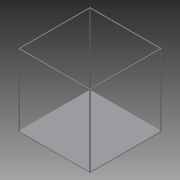
# Autodesk Inventor part: canopy
Saved by Autodesk Inventor 2014 (Build 180170000, 170)
## iProperties
Created: 2015-04-18
Part Number: canopy
Material: Generic
Document SubType Name: Modeling
Designer: Gus
Density: 1 g/cm^3
Appearance: Default
Author: Gus
Autodesk Inventor part; units mm, degrees
ref_plane "YZ Plane" through (0, 0, 0) normal (1, 0, 0) x (0, 1, 0)
ref_plane "XZ Plane" through (0, 0, 0) normal (0, 1, 0) x (-1, 0, 0)
ref_plane "XY Plane" through (0, 0, 0) normal (0, 0, 1) x (1, 0, 0)
sketch "Sketch1" plane through (0, 0, 0) normal (0, 1, 0) x (-1, 0, 0)
  line L0 (0, 0) -> (3048, 0)
  line L1 (3048, 0) -> (3048, 3048)
  line L2 (3048, 3048) -> (0, 3048)
  line L3 (0, 3048) -> (0, 0)
  dimension "d0" = 3048
  dimension "d1" = 3048
  constraints: 8 end point, 2 parallel, 1 horizontal, 1 perpendicular
  measures "d0" distance of L2.end L1.end
  measures "d1" distance of L1.end L0.end
extrude "Extrusion1" add sketch "Sketch1" along normal blind 25.4
sketch "Sketch2" plane through (0, 25.4, 0) normal (0, 1, 0) x (1, 0, 0)
  line L0 (-3048, 0) -> (-3022.6, 0)
  line L1 (-3022.6, 0) -> (-3022.6, -25.4)
  line L2 (-3022.6, -25.4) -> (-3048, -25.4)
  line L3 (-3048, -25.4) -> (-3048, 0)
  line L4 (0, 0) -> (-25.4, 0)
  line L5 (-25.4, 0) -> (-25.4, -25.4)
  line L6 (-25.4, -25.4) -> (0, -25.4)
  line L7 (0, -25.4) -> (0, 0)
  line L8 (-3048, -3048) -> (-3022.6, -3048)
  line L9 (-3022.6, -3048) -> (-3022.6, -3022.6)
  line L10 (-3022.6, -3022.6) -> (-3048, -3022.6)
  line L11 (-3048, -3022.6) -> (-3048, -3048)
  line L12 (0, -3048) -> (-25.4, -3048)
  line L13 (-25.4, -3048) -> (-25.4, -3022.6)
  line L14 (-25.4, -3022.6) -> (0, -3022.6)
  line L15 (0, -3022.6) -> (0, -3048)
  dimension "d4" = 25.4
  dimension "d5" = 25.4
  dimension "d6" = 25.4
  dimension "d7" = 25.4
  dimension "d8" = 25.4
  dimension "d9" = 25.4
  dimension "d10" = 25.4
  dimension "d11" = 25.4
  constraints: 32 end point, 8 parallel, 4 horizontal, 4 perpendicular
  measures "d4" distance of L1.end L2.end
  measures "d5" distance of L0.end L1.end
  measures "d6" distance of L6.end L5.end
  measures "d7" distance of L5.end L4.end
  measures "d8" distance of L10.end L9.end
  measures "d9" distance of L9.end L8.end
  measures "d10" distance of L13.end L14.end
  measures "d11" distance of L12.end L13.end
extrude "Extrusion2" add sketch "Sketch2" along normal blind 3048
sketch "Sketch3" plane through (0, 0, 3048) normal (1, 0, 0) x (0, 0, -1)
  line L0 (3022.6, 25.4) -> (3022.6, 3073.4) projected
  line L1 (0, 3073.4) -> (3022.6, 3073.4)
  line L2 (3022.6, 3073.4) -> (3022.6, 3048)
  line L3 (3022.6, 3048) -> (0, 3048)
  line L4 (0, 3048) -> (0, 3073.4)
  dimension "d14" = 25.4
  constraints: 8 end point, 2 parallel, 1 horizontal, 1 perpendicular, 1 point on line
  measures "d14" distance of L1.end L2.end
extrude "Extrusion3" add sketch "Sketch3" against normal blind 25.4
sketch "Sketch4" plane through (-3048, 0, 3048) normal (0, 0, 1) x (1, 0, 0)
  line L0 (0, 3073.4) -> (3048, 3073.4)
  line L1 (3048, 3073.4) -> (3048, 3048)
  line L2 (3048, 3048) -> (0, 3048)
  line L3 (0, 3048) -> (0, 3073.4)
  dimension "d17" = 3048
  dimension "d18" = 25.4
  constraints: 8 end point, 2 parallel, 1 horizontal, 1 perpendicular
  measures "d17" distance of L1.end L2.end
  measures "d18" distance of L0.end L1.end
extrude "Extrusion4" add sketch "Sketch4" against normal blind 25.4
sketch "Sketch5" plane through (-3048, 0, 0) normal (-1, 0, 0) x (0, 0, 1)
  line L0 (0, 3073.4) -> (3048, 3073.4)
  line L1 (3048, 3073.4) -> (3048, 3048)
  line L2 (3048, 3048) -> (0, 3048)
  line L3 (0, 3048) -> (0, 3073.4)
  dimension "d21" = 3048
  dimension "d22" = 25.4
  constraints: 8 end point, 2 parallel, 1 horizontal, 1 perpendicular
  measures "d21" distance of L1.end L2.end
  measures "d22" distance of L0.end L1.end
extrude "Extrusion5" add sketch "Sketch5" against normal blind 25.4
sketch "Sketch6" plane through (0, 0, 0) normal (0, 0, -1) x (-1, 0, 0)
  line L0 (0, 3073.4) -> (3048, 3073.4)
  line L1 (3048, 3073.4) -> (3048, 3048)
  line L2 (3048, 3048) -> (0, 3048)
  line L3 (0, 3048) -> (0, 3073.4)
  dimension "d25" = 3048
  dimension "d26" = 25.4
  constraints: 8 end point, 2 parallel, 1 horizontal, 1 perpendicular
  measures "d25" distance of L1.end L2.end
  measures "d26" distance of L0.end L1.end
extrude "Extrusion6" add sketch "Sketch6" against normal blind 25.4
body "Solid1"
